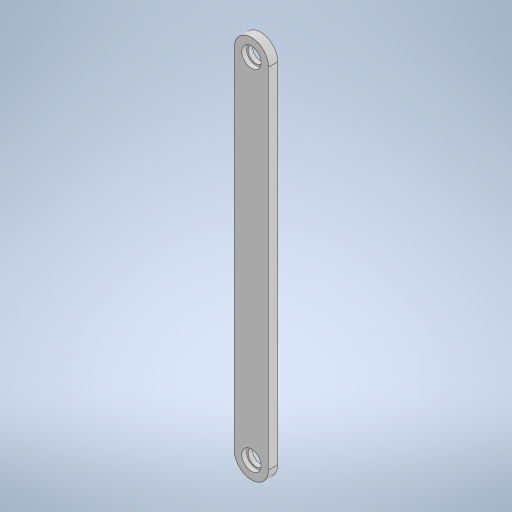
# Autodesk Inventor part: motor_holder_top
Saved by Autodesk Inventor 2024 (Build 280153000, 153)
## iProperties
Created: 2025-03-25
Part Number: motor_holder_top
Material: 一般
Document SubType Name: Modeling
Designer: 1412z
Density: 1 g/cm^3
Appearance: 既定
Author: 1412z
Autodesk Inventor part; units mm, degrees
ref_plane "YZ Plane" through (0, 0, 0) normal (1, 0, 0) x (0, 1, 0)
ref_plane "XZ Plane" through (0, 0, 0) normal (0, 1, 0) x (-1, 0, 0)
ref_plane "XY Plane" through (0, 0, 0) normal (0, 0, 1) x (1, 0, 0)
sketch "スケッチ1" plane through (0, 0, 0) normal (0, 1, 0) x (-1, 0, 0)
  point P0 (0, 0)
sketch "スケッチ2" plane through (0, 0, 0) normal (0, 0, 1) x (1, 0, 0)
  circle A0 centre (0, 0) radius 3.5
  circle A1 centre (0, 0) radius 7.5
  line L0 (0, 0) -> (0, -152.95)
  circle A2 centre (0, -152.95) radius 3.5
  circle A3 centre (0, -152.95) radius 7.5
  line L1 (7.5, -152.95) -> (7.5, 0)
  line L2 (-7.5, 0) -> (-7.5, -152.95)
  dimension "d0" = 7
  dimension "d1" = 15
  dimension "d2" = 152.95
  dimension "d3" = 7
  dimension "d4" = 15
  constraints: 6 end point, 4 centre point, 4 coincident, 4 point on circle, 2 tangent, 2 vertical
  measures "d0" diameter of A0
  measures "d1" diameter of A1
  measures "d2" distance of L0.start L0.end
  measures "d3" diameter of A2
  measures "d4" diameter of A3
extrude "押し出し1" add sketch "スケッチ2" along normal blind 4
sketch "スケッチ4" plane through (0, 0, 4) normal (0, 0, 1) x (1, 0, 0)
  arc A0 (7.5, 0) -> (-7.5, 0) centre (0, 0) ccw projected
  circle A1 centre (0, 0) radius 4.25
  circle A2 centre (0, -152.95) radius 3.5 projected
  circle A3 centre (0, -152.95) radius 4.25
  dimension "d10" = 8.5
  dimension "d11" = 8.5
  constraints: 2 centre point, 2 coincident
  measures "d10" diameter of A1
  measures "d11" diameter of A3
extrude "押し出し3" cut sketch "スケッチ4" against normal blind 2
